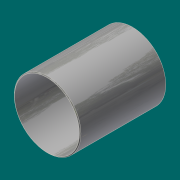
# Autodesk Inventor part: A1-19027-200-xx 34in pipe
Saved by Autodesk Inventor 2017.3 (Build 213256000, 256)
## iProperties
Created: 2019-06-26
Part Number: A1-19027-200-xx 34in pipe
Material: Steel, Mild
Document SubType Name: Modeling
Designer: Graeme_Van_Dongen
Density: 7.85 g/cm^3
Appearance: Steel
Mass: 366030 g
Surface Area: 74202.6 cm^2
Volume: 46628 cm^3
Author: Graeme_Van_Dongen
Autodesk Inventor part; units mm, degrees
ref_plane "YZ Plane" through (0, 0, 0) normal (1, 0, 0) x (0, 1, 0)
ref_plane "XZ Plane" through (0, 0, 0) normal (0, 1, 0) x (-1, 0, 0)
ref_plane "XY Plane" through (0, 0, 0) normal (0, 0, 1) x (1, 0, 0)
sketch "Sketch1" plane through (0, 0, 0) normal (0, 0, 1) x (1, 0, 0)
  circle A0 centre (0, 0) radius 431.8
  circle A1 centre (0, 0) radius 419.1
  dimension "d0" = 863.6
  dimension "d1" = 838.2
  constraints: 2 centre point, 2 coincident
  measures "d0" diameter of A0
  measures "d1" diameter of A1
extrude "Extrusion1" add sketch "Sketch1" along normal blind 1115.6125
chamfer "Chamfer1" distance 11.1125 angle 37.5 1 edges at (-431.8, 0, 0) measured on face at (-431.3, 0, 0)
chamfer "Chamfer2" distance 11.1125 angle 37.5 1 edges at (-431.8, 0, 1115.6125) measured on face at (-431.3, 0, 1115.6125)
equation "\"d7\" = d4"
equation "\"d9\" = d6"
equation "\"d4\" = 11.1125"
equation "\"d6\" = 37.5deg"
body "Solid1"
